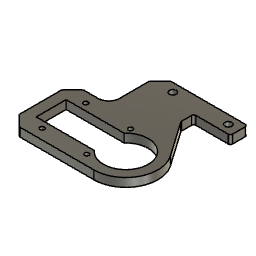
headcamera_plate_2L (Autodesk Fusion 360 design; units mm, degrees)
Autodesk Fusion 360 part; units mm, degrees
note: some values were not read from the file. Set by a fixed rule: which sketch regions a step uses; the direction of a hole.
sketch "スケッチ1" plane through (0, 0, 0) normal (0, 0, 1) x (1, 0, 0)
  line L0 (-35, -15) -> (0, -15)
  circle A0 centre (0, 0) radius 15
  line L1 (12.2873, 8.6036) -> (0.8064, 25)
  circle A1 centre (0, 0) radius 10.5
  line L2 (-29, 10.25) -> (-8, 10.25)
  line L3 (-8, 10.25) -> (-8, -10.25)
  line L4 (-8, -10.25) -> (-29, -10.25)
  line L5 (-29, -10.25) -> (-29, 10.25)
  line L6 (-13, 35) -> (13, 35)
  line L7 (-35, -15) -> (-40, -10)
  line L8 (-40, -10) -> (-40, 10)
  line L9 (-23, 15) -> (-35, 15)
  line L10 (-35, 15) -> (-40, 10)
  line L11 (0.8064, 25) -> (0.8064, 31)
  line L12 (0.8064, 31) -> (18, 31)
  line L13 (18, 31) -> (18, 39)
  line L14 (18, 39) -> (-18, 39)
  line L15 (-18, 39) -> (-23, 34)
  line L16 (-23, 34) -> (-23, 15)
  line L17 (-35, 7) -> (-7.8262, 7)
  line L18 (-7.8262, 7) -> (-7.8262, -7)
  line L19 (-7.8262, -7) -> (-35, -7)
  line L20 (-35, -7) -> (-35, 7)
  point P0 (-8, 0)
  point P1 (-11.5, 0)
  point P2 (-29.7, 0)
  point P3 (18, 35)
  point P4 (-7.8262, 0)
  dimension "d1" = 30
  dimension "d2" = 55
  dimension "d3" = 35
  dimension "d6" = 21
  dimension "d7" = 8
  dimension "d8" = 21
  dimension "d9" = 20.5
  dimension "d28" = 26
  dimension "d35" = 5
  dimension "d36" = 5
  dimension "d64" = 25
  dimension "d65" = 6
  dimension "d66" = 8
  dimension "d67" = 18
  dimension "d68" = 5
  dimension "d71" = 5
  dimension "d72" = 5
  dimension "d74" = 5
  dimension "d75" = 5
  dimension "d76" = 5
  dimension "d82" = 35
  dimension "d83" = 20
  dimension "d84" = 14
  constraint horizontal L0
  constraint coincident A0.centre A1.centre
  constraint coincident L0.end A0
  constraint tangent L0 A0
  constraint coincident A0 L1.start
  constraint tangent A0 L1
  constraint horizontal L2
  constraint vertical L3
  constraint horizontal L4
  constraint vertical L5
  constraint midpoint L3 P0
  constraint horizontal A0.centre P0
  constraint vertical L8
  constraint horizontal A0.centre P1
  constraint horizontal P1 P2
  constraint vertical L11
  constraint perpendicular L11 L12
  constraint perpendicular L12 L13
  constraint perpendicular L13 L14
  constraint midpoint L13 P3
  constraint horizontal L6.end P3
  constraint horizontal L9
  constraint perpendicular L14 L16
  constraint coincident L9.start L16.end
  constraint horizontal L6
  constraint horizontal L17
  constraint vertical L18
  constraint horizontal L19
  constraint vertical L20
  constraint midpoint L18 P4
  constraint horizontal A0.centre P4
  constraint coincident A1 L17.end
  measures "d1" diameter of A0
  measures "d2" angle of L0 L1
  measures "d3" distance of L0.start L0.end
  measures "d6" diameter of A1
  measures "d7" distance of A0.centre L3
  measures "d8" distance of L3.end L4.end
  measures "d9" distance of L2.start L4.end
  measures "d28" distance of L6.start L6.end
  measures "d35" horizontal distance of L0.start L7.end
  measures "d36" vertical distance of L0.start L7.end
  measures "d64" vertical distance of L1.end A0.centre
  measures "d65" distance of L1.end L11.end
  measures "d66" distance of L12.end L13.end
  measures "d67" distance of A0.centre L13
  measures "d68" distance of L6.end L13
  measures "d71" vertical distance of L8.end L9.end
  measures "d72" horizontal distance of L8.end L9.end
  measures "d74" horizontal distance of L6.start L14.end
  measures "d75" horizontal distance of L14.end L15.end
  measures "d76" vertical distance of L14.end L15.end
  measures "d82" distance of A0.centre L20
  measures "d83" distance of L7.end L8.end
  measures "d84" distance of L17.start L19.end
extrude "押し出し1" add sketch "スケッチ1" along normal blind 4 contours L0 A0 L1 L2 L4 L5 L7 L8 L9 L10 L11 L12 L13 L14 L15 L16 L17 L19 L20 | A0 A1 L2 L3 L4 L17 L19 | A0 L4 L5 L19 | A0 L3 L4 L19 | A0 L2 L3 L17 | A0 L2 L5 L17
hole "穴1" at (-8, 10.25, 0) at (-8, -10.25, 0) at (-29, -10.25, 0) at (-29, 10.25, 0) direction (0, 0, 1) diameter 2.1 depth 10 tip angle 118
hole "穴3" at (-13, 35, 0) at (13, 35, 0) direction (0, 0, 1) diameter 3.2 depth 10 tip angle 118
fillet "フィレット4" radius 1 10 edges at (-35, -15, 2) (-40, -10, 2) (-40, 10, 2) (-35, 15, 2) (-23, 34, 2) (-18, 39, 2) (18, 39, 2) (18, 31, 2) (0.8064, 25, 2) (0.8064, 31, 2)
fillet "フィレット5" radius 5 1 edges at (-23, 15, 2)
